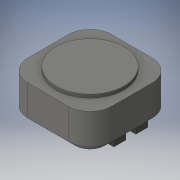
# Autodesk Inventor part: Inductor_SMD_12mm
Saved by Autodesk Inventor 2016 (Build 200138000, 138)
## iProperties
Created: 2016-09-30
Part Number: Inductor_SMD_12mm
Material: Generic
Document SubType Name: Modeling
Designer: jfixelle
Density: 1 g/cm^3
Appearance: Gray
Author: jfixelle
Autodesk Inventor part; units mm, degrees
ref_plane "YZ Plane" through (0, 0, 0) normal (1, 0, 0) x (0, 1, 0)
ref_plane "XZ Plane" through (0, 0, 0) normal (0, 1, 0) x (-1, 0, 0)
ref_plane "XY Plane" through (0, 0, 0) normal (0, 0, 1) x (1, 0, 0)
sketch "Sketch1" plane through (0, 0, 0) normal (0, 1, 0) x (-1, 0, 0)
  line L0 (6.15, 6.15) -> (-6.15, 6.15)
  line L1 (-6.15, 6.15) -> (-6.15, -6.15)
  line L2 (-6.15, -6.15) -> (6.15, -6.15)
  line L3 (6.15, -6.15) -> (6.15, 6.15)
  point P0 (0, 0)
  dimension "d0" = 12.3
  dimension "d1" = 12.3
  dimension "d2" = 6.15
  dimension "d3" = 6.15
  constraints: 8 end point, 2 parallel, 1 horizontal, 1 perpendicular
  measures "d0" distance of L2.end L0.start
  measures "d1" distance of L1.end L2.end
  measures "d2" distance from line of point (0, 0) L3
  measures "d3" distance from line of point (0, 0) L2
extrude "Extrusion1" add sketch "Sketch1" along normal blind 5.5
fillet "Fillet1" radius 3.175 4 edges at (6.15, 2.75, 6.15) (-6.15, 2.75, 6.15) (6.15, 2.75, -6.15) (-6.15, 2.75, -6.15)
sketch "Sketch2" plane through (0, 5.5, 0) normal (0, 1, 0) x (1, 0, 0)
  circle A0 centre (0, 0) radius 4.9967
  constraints: 1 centre point, 1 coincident
extrude "Extrusion2" add sketch "Sketch2" along normal blind 0.5
chamfer "Chamfer1" distance 1 angle 45 8 edges at (0, 0, 6.15) (5.2201, 0, 5.2201) (6.15, 0, 0) (5.2201, 0, -5.2201) (0, 0, -6.15) (-5.2201, 0, -5.2201) (-6.15, 0, 0) (-5.2201, 0, 5.2201)
sketch "Sketch3" plane through (0, 0, 0) normal (0, -1, 0) x (1, 0, 0)
  line L0 (-6, -2.5) -> (-3.8, -2.5)
  line L1 (-3.8, -2.5) -> (-3.8, -0.7387)
  line L2 (-3.8, -0.7387) -> (-6, -0.7387)
  line L3 (-6, -0.7387) -> (-6, -2.5)
  point P0 (0, 0)
  dimension "d12" = 2.5
  dimension "d13" = 3.8
  dimension "d16" = 6
  constraints: 8 end point, 2 parallel, 1 horizontal, 1 perpendicular
  measures "d12" distance from line of point (0, 0) L0
  measures "d13" distance from line of point (0, 0) L1
  measures "d16" distance from line of point (0, 0) L3
extrude "Extrusion3" add sketch "Sketch3" against normal blind 1
mirror "Mirror1" about plane through (0, 0, 0) normal (0, 0, 1) of "Extrusion3"
mirror "Mirror2" about plane through (0, 0, 0) normal (1, 0, 0) of "Extrusion3", "Mirror1"
body "Solid1"
